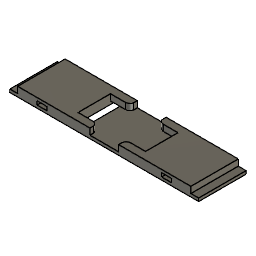
Canal - middle plate v8 (Autodesk Fusion 360 design; units mm, degrees)
Autodesk Fusion 360 part; units mm, degrees
sketch "Esquisse1" plane through (0, 0, 0) normal (0, 0, 1) x (1, 0, 0)
  line L0 (9.4, 40) -> (70, 40)
  line L1 (70, 40) -> (70, 24.75)
  line L2 (70, 24.75) -> (9.4, 24.75)
  line L3 (9.4, 24.75) -> (9.4, 40)
  dimension "d1" = 60.6
  dimension "d2" = 15.25
  constraint horizontal L0
  constraint vertical L1
  constraint horizontal L2
  constraint vertical L3
  measures "d1" distance of L1 L3
  measures "d2" distance of L0 L2
extrude "Extrusion1" add sketch "Esquisse1" along normal blind 3
sketch "Esquisse3" plane through (0, 0, 3) normal (0, 0, 1) x (-1, 0, 0)
  line L0 (-9.4, -24.75) -> (-70, -24.75)
  line L1 (-70, -24.75) -> (-70, -40)
  line L2 (-70, -40) -> (-9.4, -40)
  line L3 (-9.4, -40) -> (-9.4, -24.75)
  line L4 (-28.875, -40.2) -> (-50.525, -40.2)
  line L5 (-50.525, -40.2) -> (-50.525, -24.55)
  line L6 (-50.525, -24.55) -> (-28.875, -24.55)
  line L7 (-28.875, -24.55) -> (-28.875, -40.2)
  line L8 (-9.4, -32.375) -> (-70, -32.375) construction
  line L9 (-39.7, -40) -> (-39.7, -24.75) construction
  line L10 (-50.525, -27.175) -> (-45.775, -27.175)
  line L11 (-44.275, -25.675) -> (-44.275, -24.55)
  line L12 (-35.125, -24.55) -> (-35.125, -25.675)
  line L13 (-28.875, -37.575) -> (-33.625, -37.575)
  line L14 (-35.125, -39.075) -> (-35.125, -40.2)
  line L15 (-50.525, -37.575) -> (-45.775, -37.575)
  line L16 (-44.275, -39.075) -> (-44.275, -40.2)
  line L17 (-33.625, -27.175) -> (-28.875, -27.175)
  arc A0 (-45.775, -27.175) -> (-44.275, -25.675) centre (-45.775, -25.675) ccw
  arc A1 (-35.125, -25.675) -> (-33.625, -27.175) centre (-33.625, -25.675) ccw
  arc A2 (-33.625, -37.575) -> (-35.125, -39.075) centre (-33.625, -39.075) ccw
  arc A3 (-44.275, -39.075) -> (-45.775, -37.575) centre (-45.775, -39.075) ccw
  dimension "d8" = 21.65
  dimension "d9" = 15.65
  dimension "d30" = 10.4
  dimension "d31" = 10.4
  dimension "d32" = 9.15
  dimension "d33" = 9.15
  dimension "d34" = 1.5
  constraint horizontal L4
  constraint vertical L5
  constraint horizontal L6
  constraint vertical L7
  constraint midpoint L3 L8.start
  constraint midpoint L1 L8.end
  constraint midpoint L2 L9.start
  constraint midpoint L0 L9.end
  constraint symmetric L5 L7 L9
  constraint symmetric L0 L2 L8
  constraint symmetric L4 L6 L8
  constraint coincident L5 L10.start
  constraint perpendicular L5 L10
  constraint coincident L6 L11.end
  constraint perpendicular L6 L11
  constraint coincident L6 L12.start
  constraint perpendicular L6 L12
  constraint coincident L7 L13.start
  constraint perpendicular L7 L13
  constraint coincident L4 L14.end
  constraint perpendicular L4 L14
  constraint coincident L5 L15.start
  constraint perpendicular L5 L15
  constraint coincident L4 L16.end
  constraint perpendicular L4 L16
  constraint coincident L7 L17.end
  constraint perpendicular L7 L17
  constraint symmetric L8 L13 L17
  constraint symmetric L8 L10 L15
  constraint symmetric L9 L11 L12
  constraint symmetric L9 L14 L16
  constraint tangent L10 A0
  constraint tangent L11 A0
  constraint tangent L12 A1
  constraint tangent L17 A1
  constraint equal A0 A1
  constraint tangent L13 A2
  constraint tangent L14 A2
  constraint equal A0 A2
  constraint tangent L15 A3
  constraint tangent L16 A3
  constraint equal A0 A3
  measures "d8" distance of L5 L7
  measures "d9" distance of L4 L6
  measures "d30" distance of L13 L17
  measures "d31" distance of L10 L15
  measures "d32" distance of L11 L12
  measures "d33" distance of L14 L16
  measures "d34" radius of A0
extrude "Extrusion3" cut sketch "Esquisse3" against normal blind 2 contours L0 L2 L5 L7 L10 L11 L12 L13 L14 L15 L16 L17 A0 A1 A2 A3 | L0 L6 L11 L12 | L2 L4 L14 L16
sketch "Esquisse4" plane through (0, 0, 1) normal (0, 0, 1) x (-1, 0, 0)
  line L0 (-50.525, -27.175) -> (-50.525, -37.575)
  line L1 (-28.875, -37.575) -> (-28.875, -27.175)
  line L2 (-28.875, -27.175) -> (-31.875, -27.175)
  line L3 (-31.875, -27.175) -> (-31.875, -39.65)
  line L4 (-31.875, -39.65) -> (-28.875, -39.65)
  line L5 (-28.875, -39.65) -> (-28.875, -27.175)
  line L6 (-50.525, -37.575) -> (-45.775, -37.575)
  line L7 (-44.275, -39.075) -> (-44.275, -40)
  line L8 (-35.125, -40) -> (-35.125, -39.075)
  line L9 (-33.625, -37.575) -> (-28.875, -37.575)
  line L10 (-28.875, -27.175) -> (-33.625, -27.175)
  line L11 (-35.125, -25.675) -> (-35.125, -24.75)
  line L12 (-44.275, -24.75) -> (-44.275, -25.675)
  line L13 (-45.775, -27.175) -> (-50.525, -27.175)
  arc A0 (-44.275, -39.075) -> (-45.775, -37.575) centre (-45.775, -39.075) ccw
  arc A1 (-33.625, -37.575) -> (-35.125, -39.075) centre (-33.625, -39.075) ccw
  arc A2 (-35.125, -25.675) -> (-33.625, -27.175) centre (-33.625, -25.675) ccw
  arc A3 (-45.775, -27.175) -> (-44.275, -25.675) centre (-45.775, -25.675) ccw
  line L14 (-44.275, -40) -> (-35.125, -40)
  line L15 (-35.125, -24.75) -> (-44.275, -24.75)
  dimension "d15" = 3
  constraint horizontal L2
  constraint vertical L3
  constraint horizontal L4
  constraint vertical L5
  constraint coincident L1.end L2.start
  measures "d15" distance of L3 L5
extrude "Extrusion4" cut sketch "Esquisse4" against normal blind 3 contours L1 L2 L3 L5 L9 L10 | L3 L4 L5 L9
sketch "Esquisse5" plane through (0, 40, 0) normal (0, 1, 0) x (-1, 0, 0)
  line L0 (-70, 0) -> (-9.4, 0)
  line L1 (-9.4, 0) -> (-9.4, 3)
  line L2 (-44.275, 3) -> (-70, 3)
  line L3 (-70, 3) -> (-70, 0)
  line L4 (-39.7, 3) -> (-39.7, 0) construction
  line L5 (-44.3, 3) -> (-35.1, 3)
  line L6 (-35.1, 3) -> (-35.1, 1)
  line L7 (-35.1, 1) -> (-44.3, 1)
  line L8 (-44.3, 1) -> (-44.3, 3)
  line L9 (-21.3, 2.1) -> (-18.1, 2.1)
  line L10 (-18.1, 2.1) -> (-18.1, 0.9)
  line L11 (-18.1, 0.9) -> (-21.3, 0.9)
  line L12 (-21.3, 0.9) -> (-21.3, 2.1)
  line L13 (-19.7, 2.1) -> (-19.7, 0.9) construction
  line L14 (-58.1, 2.1) -> (-61.3, 2.1)
  line L15 (-61.3, 2.1) -> (-61.3, 0.9)
  line L16 (-61.3, 0.9) -> (-58.1, 0.9)
  line L17 (-58.1, 0.9) -> (-58.1, 2.1)
  line L18 (-44.275, 1) -> (-44.275, 3)
  line L19 (-9.4, 3) -> (-35.125, 3)
  line L20 (-35.125, 3) -> (-35.125, 1)
  line L21 (-35.125, 1) -> (-44.275, 1)
  dimension "d18" = 9.2
  dimension "d19" = 2
  dimension "d35" = 3.2
  dimension "d36" = 1.2
  dimension "d37" = 0.9
  dimension "d38" = 20
  constraint midpoint L0 L4.end
  constraint horizontal L5
  constraint vertical L6
  constraint horizontal L7
  constraint vertical L8
  constraint coincident L2 L5.start
  constraint symmetric L4 L6 L8
  constraint horizontal L9
  constraint vertical L10
  constraint horizontal L11
  constraint vertical L12
  constraint midpoint L9 L13.start
  constraint midpoint L11 L13.end
  constraint symmetric L4 L9.start L14.start
  constraint symmetric L4 L9.end L14.end
  constraint symmetric L4 L10.end L15.end
  constraint symmetric L4 L11.end L16.end
  measures "d18" distance of L6 L8
  measures "d19" distance of L5 L7
  measures "d35" distance of L9.start L9.end
  measures "d36" distance of L9.end L10.end
  measures "d37" distance of L0 L11
  measures "d38" distance of L4 L13
extrude "Extrusion5" cut sketch "Esquisse5" against normal blind 21 contours L2 L5 L7 L8 L18 | L5 L6 L7 L19 L20 | L5 L7 L18 L20 L21 | L9 L10 L11 L12 | L14 L15 L16 L17
sketch "Esquisse6" plane through (0, 0, 3) normal (0, 0, 1) x (-1, 0, 0)
  line L0 (-44.3, -25.9477) -> (-44.3, -24.75)
  line L1 (-44.3, -24.75) -> (-70, -24.75)
  line L2 (-70, -24.75) -> (-70, -40)
  line L3 (-70, -40) -> (-44.3, -40)
  line L4 (-44.3, -40) -> (-44.3, -38.8023)
  line L5 (-50.525, -37.575) -> (-50.525, -27.175)
  line L6 (-70, -40) -> (-67.5, -40)
  line L7 (-67.5, -40) -> (-67.5, -24.75)
  line L8 (-67.5, -24.75) -> (-70, -24.75)
  line L9 (-70, -24.75) -> (-70, -40)
  line L10 (-39.7, -39) -> (-39.7, -18) construction
  line L11 (-9.4, -24.75) -> (-9.4, -40)
  line L12 (-11.9, -24.75) -> (-9.4, -24.75)
  line L13 (-11.9, -40) -> (-11.9, -24.75)
  line L14 (-9.4, -40) -> (-11.9, -40)
  line L15 (-45.775, -37.575) -> (-50.525, -37.575)
  line L16 (-50.525, -27.175) -> (-45.775, -27.175)
  arc A0 (-44.3, -38.8023) -> (-45.775, -37.575) centre (-45.775, -39.075) ccw
  arc A1 (-45.775, -27.175) -> (-44.3, -25.9477) centre (-45.775, -25.675) ccw
  dimension "d22" = 2.5
  dimension "d23" = 30.3
  constraint horizontal L6
  constraint vertical L7
  constraint horizontal L8
  constraint vertical L9
  constraint coincident L1 L7.end
  constraint coincident L2.end L3.start
  constraint parallel L5 L10
  constraint symmetric L2.end L10 L11.end
  constraint symmetric L6.end L10 L13.start
  constraint symmetric L7.end L10 L12.start
  constraint symmetric L1.end L10 L11.start
  measures "d22" distance of L7 L9
  measures "d23" distance of L9 L10
extrude "Extrusion6" cut sketch "Esquisse6" against normal blind 2 contours L1 L2 L3 L6 L7 L8 L9 | L11 L12 L13 L14
